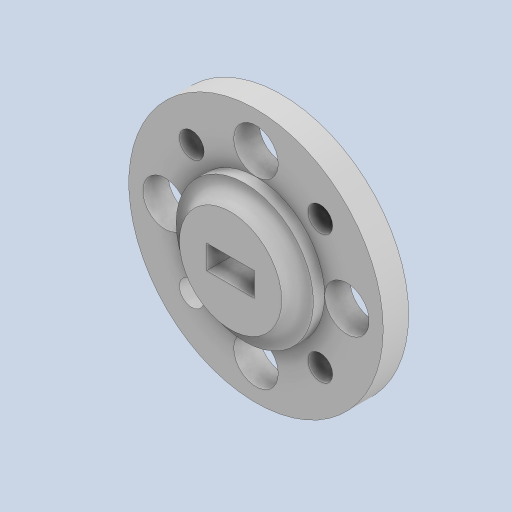
# Autodesk Inventor part: Hohlleiter-EndflanschV4
Saved by Autodesk Inventor 2023.2 (Build 272271000, 271)
## iProperties
Created: 2023-01-30
Part Number: Hohlleiter-EndflanschV4
Material: Generisch
Document SubType Name: Modeling
Designer: Nils Bade
Density: 1 g/cm^3
Appearance: Vorgabe
Author: Nils Bade
Autodesk Inventor part; units mm, degrees
ref_plane "YZ Plane" through (0, 0, 0) normal (1, 0, 0) x (0, 1, 0)
ref_plane "XZ Plane" through (0, 0, 0) normal (0, 1, 0) x (-1, 0, 0)
ref_plane "XY Plane" through (0, 0, 0) normal (0, 0, 1) x (1, 0, 0)
sketch "Endflansch" plane through (0, 0, 0) normal (0, 0, 1) x (1, 0, 0)
  circle A0 centre (0, 0) radius 10
  line L0 (0, 14) -> (0, -14) construction
  line L1 (-14, 0) -> (14, 0) construction
  line L2 (-1.8795, -0.94) -> (1.8795, -0.94)
  line L3 (1.8795, -0.94) -> (1.8795, 0.94)
  line L4 (1.8795, 0.94) -> (-1.8795, 0.94)
  line L5 (-1.8795, 0.94) -> (-1.8795, -0.94)
  line L6 (-1.8795, -0.94) -> (1.8795, 0.94) construction
  line L7 (1.8795, -0.94) -> (-1.8795, 0.94) construction
  circle A1 centre (0, 7.145) radius 1.75
  line L8 (0, 0) -> (9.8265, 9.8265) construction
  circle A2 centre (5.0523, 5.0523) radius 0.975
  circle A3 centre (0, 0) radius 7.145 construction
  circle A4 centre (0, 0) radius 3.865
  circle A5 centre (-7.145, 0) radius 1.75
  circle A6 centre (-5.0523, 5.0523) radius 0.975
  circle A7 centre (0, -7.145) radius 1.75
  circle A8 centre (-5.0523, -5.0523) radius 0.975
  circle A9 centre (7.145, 0) radius 1.75
  circle A10 centre (5.0523, -5.0523) radius 0.975
  dimension "d1" = 20
  dimension "d3" = 1.88
  dimension "d4" = 3.759
  dimension "d5" = 90
  dimension "d7" = 3.5
  dimension "d8" = 45
  dimension "d9" = 1.95
  dimension "d10" = 7.145
  dimension "d14" = 360
  dimension "d20" = 7.73
  constraints: 14 end point, 11 centre point, 3 coincident, 2 midpoint, 2 parallel, 2 point on circle, 2 point on line, 1 perpendicular, 17 other
  measures "d1" diameter of A0
  measures "d3" distance of L2.end L3.end
  measures "d4" distance between parallel lines of L5 L3
  measures "d5" angle of L1 L3
  measures "d7" diameter of A1
  measures "d8" angle of L1 L8
  measures "d9" diameter of A2
  measures "d10" radius of A3
  measures "d20" diameter of A4
extrude "Extrusion1" add sketch "Endflansch" along normal blind 2 contours A0 | A4
extrude "Extrusion2" add sketch "Endflansch" along normal blind 2 from surface at 2 contours A4
sketch "Skizze2" plane through (0, 0, 0) normal (0, 1, 0) x (-1, 0, 0)
  line L0 (3.865, 4) -> (3.865, 2) projected
  line L1 (3.865, 2) -> (5.395, 2) projected
  line L2 (5.395, 2) -> (5.395, 0) projected
  line L3 (5.395, 0) -> (1.8795, 0) projected
  line L4 (1.8795, 0) -> (1.8795, 4) projected
  line L5 (1.8795, 4) -> (3.865, 4) projected
  line L6 (-1.8795, 4) -> (-1.8795, 0) projected
  line L7 (-1.8795, 0) -> (-5.395, 0) projected
  line L8 (-5.395, 0) -> (-5.395, 2) projected
  line L9 (-5.395, 2) -> (-3.865, 2) projected
  line L10 (-3.865, 2) -> (-3.865, 4) projected
  line L11 (-3.865, 4) -> (-1.8795, 4) projected
  line L12 (10, 0) -> (8.895, 0) projected
  line L13 (8.895, 0) -> (8.895, 2) projected
  line L14 (8.895, 2) -> (10, 2) projected
  line L15 (10, 2) -> (10, 0) projected
  line L16 (-8.895, 0) -> (-10, 0) projected
  line L17 (-10, 0) -> (-10, 2) projected
  line L18 (-10, 2) -> (-8.895, 2) projected
  line L19 (-8.895, 2) -> (-8.895, 0) projected
  line L20 (0, -1.16) -> (0, 6.96) construction
  circle A0 centre (-5, 3.8) radius 1
  line L21 (-3.865, 4) -> (-4.0202, 4)
  line L22 (-3.865, 2) -> (-3.865, 4) construction
  line L23 (-8.895, 2) -> (-5.395, 2) construction
  line L24 (-5.395, 2) -> (-5.395, 2.8813)
  point P0 (0, 0)
  dimension "d21" = 2
  dimension "d22" = 5
  dimension "d28" = 0.2
  constraints: 4 end point, 2 point on circle, 1 centre point, 1 perpendicular, 1 vertical
  measures "d21" diameter of A0
  measures "d22" distance from line of L20 A0.centre
  measures "d28" distance from line of A0.centre L11
revolve "Umdrehung1" add sketch "Skizze2" angle 360 about axis through (0, 0, -10) along (0, 0, 1) contours L10 L9 L24 A0 L21
extrude "Extrusion3" [suppressed]
equation "\"d3\" = Hohlleiter_b"
equation "\"d4\" = Hohlleiter_h"
equation "\"d7\" = Bohrung_IHF_Schraube"
equation "\"d9\" = Bohrung_IHF_Passstift"
equation "\"d20\" = Hohlleiter_Erhebung_d"
equation "\"Hohlleiter_h\" = 3.759"
equation "\"Hohlleiter_b\" = 1.88"
equation "\"Hohlleiter_Orientation\" = 0"
equation "\"Bohrung_IHF_Schraube\" = 3.5"
equation "\"Bohrung_IHF_Passstift\" = 1.95"
equation "\"Hohlleiter_Erhebung_d\" = 7.73"
